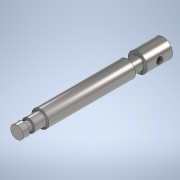
# Autodesk Inventor part: 09.TornilloSinFin.LPSM
Saved by Autodesk Inventor 2021 (Build 250183000, 183)
## iProperties
Created: 2020-10-13
Part Number: 09.TornilloSinFin.LPSM
Material: Steel, Alloy
Document SubType Name: Modeling
Designer: Quetzali
Density: 7.73 g/cm^3
Appearance: Semi-Polished
Author: Quetzali
Autodesk Inventor part; units mm, degrees
ref_plane "YZ Plane" through (0, 0, 0) normal (1, 0, 0) x (0, 1, 0)
ref_plane "XZ Plane" through (0, 0, 0) normal (0, 1, 0) x (-1, 0, 0)
ref_plane "XY Plane" through (0, 0, 0) normal (0, 0, 1) x (1, 0, 0)
sketch "Sketch1" plane through (0, 0, 0) normal (0, 0, 1) x (1, 0, 0)
  circle A0 centre (0, 0) radius 8
  dimension "d0" = 16
  constraints: 1 centre point, 1 coincident
  measures "d0" diameter of A0
extrude "Extrusion1" add sketch "Sketch1" along normal blind 82
sketch "Sketch2" plane through (0, 0, 82) normal (0, 0, 1) x (1, 0, 0)
  circle A0 centre (0, 0) radius 6
  dimension "d4" = 12
  constraints: 1 centre point, 1 coincident
  measures "d4" diameter of A0
extrude "Extrusion2" add sketch "Sketch2" along normal blind 11
sketch "Sketch3" plane through (0, 0, 93) normal (0, 0, 1) x (1, 0, 0)
  circle A0 centre (0, 0) radius 4
  dimension "d7" = 8
  constraints: 1 centre point, 1 coincident
  measures "d7" diameter of A0
extrude "Extrusion3" add sketch "Sketch3" along normal blind 5
sketch "Sketch4" plane through (0, 0, 98) normal (0, 0, 1) x (1, 0, 0)
  circle A0 centre (0, 0) radius 6
  dimension "d10" = 12
  constraints: 1 centre point, 1 coincident
  measures "d10" diameter of A0
extrude "Extrusion4" add sketch "Sketch4" along normal blind 6
sketch "Sketch5" plane through (0, 0, 0) normal (0, 0, -1) x (-1, 0, 0)
  circle A0 centre (0, 0) radius 6
  dimension "d13" = 12
  constraints: 1 centre point, 1 coincident
  measures "d13" diameter of A0
extrude "Extrusion5" add sketch "Sketch5" along normal blind 10
sketch "Sketch6" plane through (0, 0, -10) normal (0, 0, -1) x (-1, 0, 0)
  circle A0 centre (0, 0) radius 9
  dimension "d16" = 18
  constraints: 1 centre point, 1 coincident
  measures "d16" diameter of A0
extrude "Extrusion6" add sketch "Sketch6" along normal blind 24
sketch "Sketch7" plane through (0, 0, 0) normal (1, 0, 0) x (0, 1, 0)
  line L0 (-9, -10) -> (9, -10) projected
  line L1 (-9, -34) -> (9, -34) projected
  line L2 (-9, -10) -> (9, -34)
  line L3 (9, -10) -> (-9, -34)
  circle A0 centre (0, -22) radius 3
  point P0 (0, 0)
  dimension "d19" = 6
  constraints: 4 end point, 1 centre point, 1 midpoint
  measures "d19" diameter of A0
extrude "Extrusion7" cut sketch "Sketch7" against normal mid plane 24 contours A0 L3 L2 | L2 L3 A0 | A0 L2 L3 | L2 A0 L3
body "Solid1"
